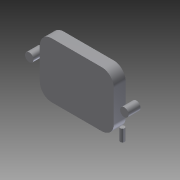
# Autodesk Inventor part: AC entry module
Saved by Autodesk Inventor 2012 (Build 160160000, 160)
## iProperties
Created: 2017-06-15
Part Number: AC entry module
Material: Default
Document SubType Name: Modeling
Designer: Brandon
Density: 1 g/cm^3
Author: Brandon
Autodesk Inventor part; units mm, degrees
ref_plane "YZ Plane" through (0, 0, 0) normal (1, 0, 0) x (0, 1, 0)
ref_plane "XZ Plane" through (0, 0, 0) normal (0, 1, 0) x (-1, 0, 0)
ref_plane "XY Plane" through (0, 0, 0) normal (0, 0, 1) x (1, 0, 0)
sketch "Sketch1" plane through (0, 0, 0) normal (0, 0, 1) x (1, 0, 0)
  line L0 (-15.55, 27.65) -> (15.55, 27.65)
  line L1 (15.55, 27.65) -> (15.55, 4.35)
  line L2 (15.55, 4.35) -> (-15.55, 4.35)
  line L3 (-15.55, 4.35) -> (-15.55, 27.65)
  circle A0 centre (20, 16) radius 1.8
  circle A1 centre (-20, 16) radius 1.8
  point P0 (0, 0)
  dimension "d0" = 23.3
  dimension "d1" = 31.1
  dimension "d3" = 15.55
  dimension "d4" = 40
  dimension "d5" = 20
  dimension "d6" = 3.6
  dimension "d7" = 3.6
  dimension "d10" = 16
  dimension "d23" = 16
  dimension "d24" = 27.65
  constraints: 8 end point, 2 centre point, 2 parallel, 1 horizontal, 1 perpendicular
  measures "d0" distance of L2.end L0.start
  measures "d1" distance of L0.start L0.end
  measures "d3" distance from line of point (0, 0) L1
  measures "d4" distance of A0.centre A1.centre
  measures "d5" horizontal distance of point (0, 0) A1.centre
  measures "d6" diameter of A0
  measures "d7" diameter of A1
  measures "d10" vertical distance of point (0, 0) A1.centre
  measures "d23" vertical distance of point (0, 0) A0.centre
  measures "d24" distance from line of point (0, 0) L0
extrude "Extrusion1" add sketch "Sketch1" along normal blind 5
fillet "Fillet1" radius 5 1 edges at (15.55, 27.65, 2.5)
fillet "Fillet2" radius 5 1 edges at (-15.55, 27.65, 2.5)
fillet "Fillet3" radius 5 1 edges at (15.55, 4.35, 2.5)
fillet "Fillet4" radius 5 1 edges at (-15.55, 4.35, 2.5)
sketch "Sketch2" plane through (0, 0, 0) normal (0, 1, 0) x (-1, 0, 0)
  circle A0 centre (0, -5.1575) radius 0.9
  circle A1 centre (-8.9999, -5.196) radius 0.9
  circle A2 centre (9, -5.1848) radius 0.9
  point P0 (0, 0)
  dimension "d17" = 1.8
  dimension "d18" = 1.8
  dimension "d19" = 9
  dimension "d20" = 9
  constraints: 3 centre point
  measures "d17" diameter of A0
  measures "d18" diameter of A1
  measures "d19" distance of A0.centre A1.centre
  measures "d20" distance of A0.centre A2.centre
extrude "Extrusion2" add sketch "Sketch2" against normal blind 5
equation "\"d3\" = 0.5 * d1"
equation "\"d5\" = 0.5 * d4"
body "Solid1"
